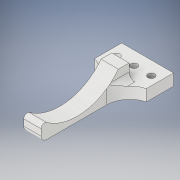
# Autodesk Inventor part: BottomBracket
Saved by Autodesk Inventor 2018 (Build 220112000, 112)
## iProperties
Created: 2019-04-14
Part Number: BottomBracket
Material: Generic
Document SubType Name: Modeling
Designer: anirudh
Density: 1 g/cm^3
Appearance: White
Author: anirudh
Autodesk Inventor part; units mm, degrees
ref_plane "YZ Plane" through (0, 0, 0) normal (1, 0, 0) x (0, 1, 0)
ref_plane "XZ Plane" through (0, 0, 0) normal (0, 1, 0) x (-1, 0, 0)
ref_plane "XY Plane" through (0, 0, 0) normal (0, 0, 1) x (1, 0, 0)
sketch "Sketch1" plane through (0, 0, 0) normal (1, 0, 0) x (0, 1, 0)
  arc A0 (-20.4823, 19.925) -> (-17.392, -22.6726) centre (0, 0) ccw
  line L0 (-24.892, 0) -> (-9.892, 0) construction
  line L1 (-24.892, -28.575) -> (-24.892, -43.575)
  line L2 (-24.892, -43.575) -> (-31.242, -43.575)
  line L3 (-31.242, -43.575) -> (-31.242, 19.925)
  line L4 (-31.242, 19.925) -> (-20.4823, 19.925)
  line L5 (-24.892, -28.575) -> (-17.392, -28.575)
  line L6 (-17.392, -28.575) -> (-17.392, -22.6726)
  dimension "d0" = 57.15
  dimension "d7" = 15
  dimension "d8" = 6.35
  dimension "d9" = 63.5
  dimension "d10" = 7.5
  constraints: 14 end point, 4 perpendicular, 2 point on circle, 1 centre point, 1 coincident, 1 horizontal
  measures "d0" diameter of A0
  measures "d7" distance of L1.start L1.end
  measures "d8" distance of L1.end L2.end
  measures "d9" distance of L2.end L3.end
  measures "d10" distance of L1.start L5.end
extrude "Extrusion1" add sketch "Sketch1" along normal blind 9.525
sketch "Sketch2" plane through (0, -24.892, -28.575) normal (0, 1, 0) x (1, 0, 0)
  line L0 (0, 0) -> (0, 15) projected
  line L1 (0, 0) -> (9.525, 0) projected
  circle A0 centre (4.7625, 7.5) radius 1.85
  point P0 (0, -28.575)
  point P1 (9.525, 15)
  dimension "d13" = 3.7
  constraints: 1 centre point
  measures "d13" diameter of A0
extrude "Extrusion2" cut sketch "Sketch2" against normal blind 25.4
sketch "Sketch3" plane through (0, -24.892, -28.575) normal (0, 1, 0) x (1, 0, 0)
  line L0 (0, 0) -> (0, 15) projected
  line L1 (0, 15) -> (-9.525, 15)
  line L2 (-9.525, 15) -> (-9.525, 0)
  line L3 (-9.525, 0) -> (0, 0)
  line L4 (0, 0) -> (0, 15)
  line L5 (9.525, 15) -> (19.05, 15)
  line L6 (19.05, 15) -> (19.05, 0)
  line L7 (19.05, 0) -> (9.525, 0)
  line L8 (9.525, 0) -> (9.525, 15)
  line L9 (9.525, -48.5) -> (9.525, 15) projected
  circle A0 centre (-4.7625, 7.5) radius 1.85
  circle A1 centre (14.2875, 7.5) radius 1.85
  point P0 (0, -28.575)
  dimension "d16" = 9.525
  dimension "d17" = 9.525
  dimension "d18" = 3.7
  dimension "d19" = 3.7
  constraints: 16 end point, 4 parallel, 2 centre point, 2 horizontal, 2 perpendicular, 1 point on line
  measures "d16" distance of L3.end L2.end
  measures "d17" distance of L6.end L7.end
  measures "d18" diameter of A0
  measures "d19" diameter of A1
extrude "Extrusion3" add sketch "Sketch3" against normal blind 6.35
fillet "Fillet1" radius 12.7 2 edges at (9.525, -28.067, -28.575) (0, -28.067, -28.575)
fillet "Fillet2" radius 3.175 2 edges at (9.525, -24.892, -22.4266) (0, -24.892, -22.4266)
fillet "Fillet3" radius 3.175 1 edges at (4.7625, -31.242, 19.925)
fillet "Fillet4" radius 1.905 1 edges at (4.7625, -20.4823, 19.925)
body "Solid1"
